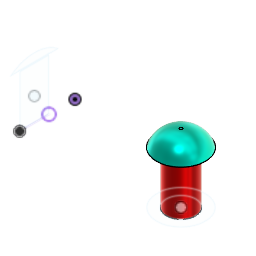
Blocker (Autodesk Fusion 360 design; units mm, degrees)
part number: 2026-05-25-19-40-37-466
Autodesk Fusion 360 part; units mm, degrees
sketch "Sketch1" plane through (0, 0, 0) normal (0, 0, 1) x (1, 0, 0)
  circle A0 centre (45, -12.4728) radius 4.5
  circle A1 centre (45, -12.4728) radius 7.5
  dimension "d3" = 9
  dimension "d5" = 45
  dimension "d6" = 12.4728
  dimension "d13" = 15
  constraint concentric A0 A1
  measures "d3" diameter of A0
  measures "d5" horizontal distance of origin A0.centre
  measures "d6" vertical distance of origin A0.centre
  measures "d13" diameter of A1
sketch "Sketch2" plane through (0, 0, 0) normal (1, 0, 0) x (0, 1, 0)
  line L0 (-7.9728, 0) -> (-16.9728, 0)
  line L1 (-16.9728, 0) -> (-7.9728, 0)
  line L2 (-7.9728, 0) -> (-7.9728, 16)
  line L3 (-7.9728, 16) -> (-16.9728, 16)
  line L4 (-16.9728, 16) -> (-16.9728, 0)
  line L5 (-19.9728, 16) -> (-4.9728, 16)
  arc A0 (-4.9728, 16) -> (-19.9728, 16) centre (-12.4728, 7.0871) ccw
  dimension "d7" = 16
  dimension "d8" = 3
  dimension "d9" = 15
  dimension "d10" = 16
  dimension "d11" = 7.9728
  dimension "d12" = 11.6486
  constraint horizontal L1
  constraint vertical L2
  constraint horizontal L3
  constraint vertical L4
  constraint coincident L0.end L1.start
  constraint perpendicular L4 L5
  measures "d7" distance of L0.end L3.end
  measures "d8" distance of L3.end L5.start
  measures "d9" distance of L5.start L5.end
  measures "d10" vertical distance of L0.start L5.end
  measures "d11" distance of origin L0.start
  measures "d12" radius of A0
extrude "Extrude1" add sketch "Sketch1" along normal blind 16 contours A0
extrude "Extrude2" add sketch "Sketch1" along normal blind 5 from surface at 16 contours A0 | A1
fillet "Fillet1" radius 7.5 1 edges at (38.0075, -15.1849, 21)
